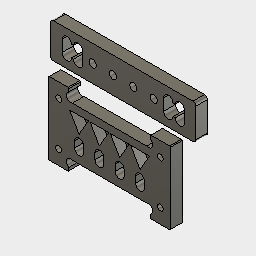
5mm_deep_thread_testx2x4 (Autodesk Fusion 360 design; units mm, degrees)
Autodesk Fusion 360 part; units mm, degrees
note: some values were not read from the file. Set by a fixed rule: which sketch regions a step uses.
sketch "Sketch1" plane through (0, 0, 0) normal (0, 0, 1) x (1, 0, 0)
  line L0 (42, 17) -> (-42, 17)
  line L1 (-42, 17) -> (-42, -17)
  line L2 (-42, -17) -> (42, -17)
  line L3 (42, -17) -> (42, 17)
  line L4 (42, 17) -> (-42, -17) construction
  line L5 (-42, 17) -> (42, -17) construction
  line L6 (-27.5, 12) -> (-14.5, 12)
  line L7 (-14.5, 12) -> (-21, 0.7417)
  line L8 (-21, 0.7417) -> (-27.5, 12)
  line L9 (-21, 12) -> (-21, 17) construction
  line L10 (-42, 17) -> (-28, 17)
  line L11 (-28, 17) -> (-28, 25)
  line L12 (-28, 25) -> (-42, 25)
  line L13 (-42, 25) -> (-42, 17)
  line L14 (-21, 0.7417) -> (-21, 8.5)
  line L15 (-13.5, 12) -> (-0.5, 12)
  line L16 (-7, 0.7417) -> (-13.5, 12)
  line L17 (-0.5, 12) -> (-7, 0.7417)
  line L18 (0.5, 12) -> (13.5, 12)
  line L19 (7, 0.7417) -> (0.5, 12)
  line L20 (13.5, 12) -> (7, 0.7417)
  line L21 (14.5, 12) -> (27.5, 12)
  line L22 (21, 0.7417) -> (14.5, 12)
  line L23 (27.5, 12) -> (21, 0.7417)
  line L24 (42, 17) -> (28, 17)
  line L25 (28, 17) -> (28, 25)
  line L26 (28, 25) -> (42, 25)
  line L27 (42, 25) -> (42, 17)
  line L28 (21, 12) -> (21, 17)
  line L29 (0, 0) -> (-42, 0) construction
  line L30 (-42, -17) -> (-28, -17)
  line L31 (-28, -17) -> (-28, -25)
  line L32 (-28, -25) -> (-42, -25)
  line L33 (28, -25) -> (42, -25)
  line L34 (28, -17) -> (28, -25)
  line L35 (42, -25) -> (42, -17)
  line L36 (-42, -25) -> (-42, -17)
  line L37 (-24.05, -4.65) -> (-24.05, -8.95)
  arc A0 (-24.05, -8.95) -> (-17.95, -8.95) centre (-21, -8.95) ccw
  line L38 (-17.95, -8.95) -> (-17.95, -4.65)
  arc A1 (-17.95, -4.65) -> (-24.05, -4.65) centre (-21, -4.65) ccw
  line L39 (-21, -4.65) -> (-21, -8.95) construction
  line L40 (-21, -12) -> (-21, -17)
  arc A2 (-3.95, -4.65) -> (-10.05, -4.65) centre (-7, -4.65) ccw
  line L41 (-10.05, -4.65) -> (-10.05, -8.95)
  line L42 (-3.95, -8.95) -> (-3.95, -4.65)
  line L43 (-7, -4.65) -> (-7, -8.95) construction
  arc A3 (-10.05, -8.95) -> (-3.95, -8.95) centre (-7, -8.95) ccw
  arc A4 (10.05, -4.65) -> (3.95, -4.65) centre (7, -4.65) ccw
  line L44 (3.95, -4.65) -> (3.95, -8.95)
  line L45 (10.05, -8.95) -> (10.05, -4.65)
  line L46 (7, -4.65) -> (7, -8.95) construction
  arc A5 (3.95, -8.95) -> (10.05, -8.95) centre (7, -8.95) ccw
  arc A6 (24.05, -4.65) -> (17.95, -4.65) centre (21, -4.65) ccw
  line L47 (17.95, -4.65) -> (17.95, -8.95)
  line L48 (24.05, -8.95) -> (24.05, -4.65)
  line L49 (21, -4.65) -> (21, -8.95) construction
  arc A7 (17.95, -8.95) -> (24.05, -8.95) centre (21, -8.95) ccw
  point P0 (-7, -12)
  point P1 (7, -12)
  point P2 (21, -12)
  dimension "d3" = 5
  dimension "d4" = 13
  dimension "d5" = 8
  dimension "d6" = 14
  dimension "d17" = 7
  dimension "d22" = 14
  dimension "d23" = 0
  dimension "d24" = 7
  dimension "d35" = 4.3
  dimension "d36" = 5
  dimension "d37" = 3.05
  dimension "d38" = 7
  dimension "d39" = 50
  dimension "d42" = 14
  dimension "d43" = 0
  dimension "d44" = 84
  measures "d3" distance of L0 L6
  measures "d4" distance of L6.start L6.end
  measures "d5" distance of L0.end L12.end
  measures "d6" distance of L0.end L10.end
  measures "d17" distance of L9.end L11
  measures "d24" distance of L25 L28.end
  measures "d35" distance of A1.centre A0.centre
  measures "d36" distance of L40.start L40.end
  measures "d37" radius of A1
  measures "d38" distance of L31 L40
  measures "d39" distance of L12 L32
  measures "d44" distance of L12.end L26.end
extrude "Extrude1" add sketch "Sketch1" along normal blind 8 makes body 1
extrude "Extrude2" add sketch "Sketch1" along normal blind 1.5 contours L6 L7 L8 | L15 L16 L17 | L18 L19 L20 | L21 L22 L23 | L37 A0 L38 A1 | A2 L41 L42 A3 | A4 L44 L45 A5 | A6 L47 L48 A7 bodies 1
sketch "Sketch2" plane through (0, -17, 0) normal (0, -1, 0) x (1, 0, 0)
  line L0 (-28, 0) -> (28, 0)
  line L1 (28, 0) -> (28, 8)
  line L2 (28, 8) -> (-28, 8)
  line L3 (-28, 8) -> (-28, 0)
  line L4 (-50, 16) -> (50, 16)
  line L5 (50, 16) -> (50, -8)
  line L6 (50, -8) -> (-50, -8)
  line L7 (-50, -8) -> (-50, 16)
  line L8 (-42, 0) -> (-42, 8)
  line L9 (-42, 4) -> (-50, 4) construction
  line L10 (42, 0) -> (42, 8)
  line L11 (42, 4) -> (50, 4) construction
  line L12 (0, 0) -> (0, 16) construction
  circle A0 centre (-38.9, 0) radius 3.1
  line L13 (-42, 8) -> (-28, 8)
  line L14 (-28, 0) -> (-42, 0)
  line L15 (-35, 8) -> (-35, 0) construction
  circle A1 centre (-38.9, 8) radius 3.1
  circle A2 centre (-31.1, 8) radius 3.1
  circle A3 centre (-31.1, 0) radius 3.1
  line L16 (-28, 8) -> (-28, 0)
  line L17 (0, -8) -> (0, 16)
  circle A4 centre (-21, 4) radius 2.5
  line L18 (-21, 4) -> (-28, 4) construction
  circle A5 centre (-7, 4) radius 2.5
  line L19 (-7, 4) -> (-21, 4) construction
  dimension "d49" = 100
  dimension "d50" = 24
  dimension "d52" = 6.2
  dimension "d65" = 5
  dimension "d66" = 7
  dimension "d67" = 14
  measures "d49" distance of L4.start L4.end
  measures "d50" distance of L4.start L6.end
  measures "d52" diameter of A0
  measures "d65" diameter of A4
  measures "d66" distance of A4.centre L18.end
  measures "d67" distance of A5.centre A4.centre
extrude "Extrude4" add sketch "Sketch2" along normal blind 8 separate body contours L0 L2 L3 L16 L17 | L0 L2 L4 L6 L7 L8 A0 L13 L14 A1 A2 A3 L17 makes body 2
sketch "Sketch3" plane through (0, 0, 0) normal (0, 0, 1) x (1, 0, 0)
  circle A0 centre (-26.8, 19.7495) radius 3
  line L0 (-28, 17) -> (-28, 25)
  line L1 (-27.5, 12) -> (-14.5, 12)
  line L2 (28, 17) -> (-28, 17)
  line L3 (-21, 12) -> (-21, 17) construction
  line L4 (-23.5, 17) -> (-18.5, 17) construction
  line L5 (-18.5, 17) -> (-18.5, 12) construction
  line L6 (-18.5, 12) -> (-23.5, 12) construction
  line L7 (-23.5, 12) -> (-23.5, 17) construction
  line L8 (-23.5, 17) -> (-18.5, 12) construction
  line L9 (-18.5, 17) -> (-23.5, 12) construction
  point P0 (-28, 17)
  point P1 (-21, 14.5)
  dimension "d54" = 6
  dimension "d58" = 5
  dimension "d59" = 1.2
  measures "d54" diameter of A0
  measures "d58" distance of L4.start L4.end
  measures "d59" distance of A0.centre P0
extrude "Extrude3" cut sketch "Sketch3" along normal up to surface (8 mm away) contours A0 L0 | A0 L2 bodies 1
fillet "Fillet1" radius 0.5 2 edges at (-28, 25, 4) (-42, 25, 4) on bodies 1
mirror "Mirror1" about plane through (0, 0, 0) normal (1, 0, 0) of 3 faces at (-28.2678, 22.3659, 5.3333) (-28.0556, 24.7291, 2.6667) (-41.5946, 24.991, 2.6667) on bodies 1
ref_plane "WorkPlane1" through (0, 0, 4) normal (0, 1, 0) x (-1, 0, 0)
mirror "Mirror2" about plane through (0, 0, 4) normal (0, 1, 0) of 6 faces at (-28.2678, 22.3659, 5.3333) (-28.0556, 24.7291, 2.6667) (-41.5946, 24.991, 2.6667) (28.1356, 22.4359, 2.6667) (28.0556, 24.7291, 2.6667) (41.5946, 24.991, 2.6667) on bodies 1
fillet "Fillet2" radius 2 2 edges at (-50, -21, -8) (-50, -21, 16) on bodies 2
move_face "OffsetFaces1" offset -0.1 4 faces at (-42, -19.6667, 2.6667) (-28, -19.6667, 5.3333) (-34.7333, -19.6667, 0) (-35.2667, -22.3333, 8) on bodies 2
mirror "Mirror3" about plane through (0, -17, 8) normal (1, 0, 0) of bodies 2 makes body 3
combine "Combine1" operation add target body 2 tool bodies 3
copy_body "Body->Comp1" bodies 1 removing the originals makes body 4 in component "drill"
copy_body "Body->Comp2" bodies 2 removing the originals makes body 5 in component "guide"
sketch "Sketch2 (2)" plane through (0, 0, 0) normal (0, 0, 1) x (1, 0, 0) in component "drill"
  circle A0 centre (-35, 15) radius 2
  circle A1 centre (-35, -15) radius 2
  line L0 (-35, 15) -> (35, 15) construction
  line L1 (35, 15) -> (35, -15) construction
  line L2 (35, -15) -> (-35, -15) construction
  line L3 (-35, -15) -> (-35, 15) construction
  line L4 (-35, 15) -> (35, -15) construction
  line L5 (35, 15) -> (-35, -15) construction
  circle A2 centre (35, 15) radius 2
  circle A3 centre (35, -15) radius 2
  dimension "d71" = 4
  dimension "d73" = 30
  dimension "d74" = 70
  measures "d71" diameter of A0
  measures "d73" distance of A0.centre A1.centre
  measures "d74" distance of A0.centre L0.end
extrude "Extrude1'" cut sketch "Sketch2 (2)" along normal up to surface (8 mm away) bodies 4 in component "drill"
sketch "Sketch1 (2)" plane through (0, 0, 0) normal (0, 0, 1) x (1, 0, 0) in component "layout"
  line L0 (0, 0) -> (140, 0)
  line L1 (140, 0) -> (140, 120)
  line L2 (140, 120) -> (0, 120)
  line L3 (0, 120) -> (0, 0)
  dimension "d77" = 140
  dimension "d78" = 120
  measures "d77" distance of L0.start L0.end
  measures "d78" distance of L0.start L2.end
extrude "Extrude1''" add sketch "Sketch1 (2)" along normal blind 8 separate body makes body 6 in component "layout"
copy_body "Body->Comp1'" bodies 6 removing the originals makes body 7 in component "stock"
component "assembled" placed x (1, 0, 0) y (0, 1, 0) z (0, 0, 1) at (0, 0, 0)
component "layout" placed x (1, 0, 0) y (0, 1, 0) z (0, 0, 1) at (0, 0, 0)
component "drill" placed x (1, 0, 0) y (0, 1, 0) z (0, 0, 1) at (0, 0, 0) in component "assembled"
component "guide" placed x (1, 0, 0) y (0, 1, 0) z (0, 0, 1) at (0, 0, 0) in component "assembled"
component "drill" placed x (1, 0, 0) y (0, 1, 0) z (0, 0, 1) at (54.399, 41.1785, 0) in component "layout"
component "guide" placed x (1, 0, 0) y (0, 0, -1) z (0, 1, 0) at (63.8482, 84.8641, -17) in component "layout"
component "stock" placed x (1, 0, 0) y (0, 1, 0) z (0, 0, 1) at (0, 0, 0) in component "layout"
equation "d24 = d17"
equation "d37 = 6.1 mm / 2"
equation "d50 = ( 8 * 3 ) * 1 mm"
